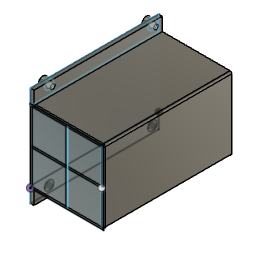
battery_holder v3 (Autodesk Fusion 360 design; units mm, degrees)
Autodesk Fusion 360 part; units mm, degrees
sketch "Sketch1" plane through (0, 0, 0) normal (0, 1, 0) x (1, 0, 0)
  line L0 (0, 0) -> (41, 0)
  line L1 (41, 0) -> (41, -41)
  line L2 (41, -41) -> (0, -41)
  line L3 (0, -41) -> (0, 0)
  line L4 (1, -1) -> (40, -1)
  line L5 (40, -1) -> (40, -40)
  line L6 (40, -40) -> (1, -40)
  line L7 (1, -40) -> (1, -1)
  line L8 (20, -40) -> (20, -1)
  line L9 (21, -40) -> (21, -1)
  line L10 (1, -21) -> (20, -21)
  line L11 (1, -20) -> (20, -20)
  line L12 (21, -21) -> (40, -21)
  line L13 (21, -20) -> (40, -20)
  dimension "d1" = 41
  dimension "d2" = 41
  dimension "d3" = 39
  dimension "d4" = 1
  dimension "d5" = 1
  dimension "d6" = 19
  dimension "d7" = 19
  dimension "d8" = 1
  dimension "d9" = 1
  dimension "d10" = 19
  dimension "d11" = 19
  constraint horizontal L0
  constraint vertical L1
  constraint horizontal L2
  constraint vertical L3
  constraint coincident L0.start L3.end
  constraint horizontal L4
  constraint vertical L5
  constraint horizontal L6
  constraint vertical L7
  constraint coincident L6 L8.start
  constraint coincident L4 L8.end
  constraint perpendicular L4 L8
  constraint coincident L6 L9.start
  constraint coincident L4 L9.end
  constraint perpendicular L4 L9
  constraint coincident L7 L10.start
  constraint coincident L8 L10.end
  constraint perpendicular L8 L10
  constraint coincident L7 L11.start
  constraint coincident L8 L11.end
  constraint perpendicular L7 L11
  constraint coincident L9 L12.start
  constraint coincident L5 L12.end
  constraint perpendicular L5 L12
  constraint coincident L9 L13.start
  constraint perpendicular L9 L13
  measures "d1" distance of L0.start L0.end
  measures "d2" distance of L0.start L2.end
  measures "d3" distance of L4.start L6.end
  measures "d4" distance of L0 L4
  measures "d5" distance of L3 L7
  measures "d6" distance of L7 L8
  measures "d7" distance of L5 L9
  measures "d8" distance of L10 L11
  measures "d9" distance of L12 L13
  measures "d10" distance of L4 L11
  measures "d11" distance of L4 L13
extrude "Extrude1" add sketch "Sketch1" along normal blind 68 contours L4 L6 L8 L9 | L7 L8 L10 L11 | L5 L9 L12 L13
extrude "Extrude2" add sketch "Sketch1" along normal blind 72
extrude "Extrude3" add sketch "Sketch1" along normal blind 2 contours L4 L7 L8 L11 | L4 L5 L9 L13 | L6 L7 L8 L10 | L5 L6 L9 L12
ref_plane "WorkPlane1" through (18, 37, 20.5) normal (1, 0, 0) x (0, 0, -1)
sketch "Sketch6" plane through (18, 0, 0) normal (1, 0, 0) x (0, 1, 0)
  line L0 (72, 40) -> (70.5, 40)
  line L1 (70.5, 40) -> (70.5, 39)
  line L2 (70.5, 39) -> (72, 40)
  line L3 (72, 1) -> (70.5, 1)
  line L4 (70.5, 1) -> (70.5, 2)
  line L5 (70.5, 2) -> (72, 1)
  constraint horizontal L0
  constraint perpendicular L0 L1
  constraint perpendicular L1 L3
  constraint perpendicular L3 L4
extrude "Extrude4" add sketch "Sketch6" along normal blind 5
fillet "Fillet1" radius 1 1 edges at (41, 36, 41)
fillet "Fillet2" radius 1 1 edges at (0, 36, 41)
fillet "Fillet3" radius 1 5 edges at (41, 0, 20) (40.7071, 0, 40.7071) (20.5, 0, 41) (0.2929, 0, 40.7071) (0, 0, 20)
fillet "Fillet4" radius 1 5 edges at (41, 36.5, 0) (40.7071, 0.2929, 0) (20.5, 0, 0) (0.2929, 0.2929, 0) (0, 36.5, 0)
sketch "Sketch8" plane through (0, 0, 0) normal (-1, 0, 0) x (0, -1, 0)
  line L0 (-72, 1) -> (-1, 1)
  line L1 (-1, 1) -> (-1, 40)
  line L2 (-1, 40) -> (-72, 40)
  line L3 (-72, 40) -> (-72, 1)
  line L4 (-72, 1) -> (0, 1)
  line L5 (0, 1) -> (0, -7.5)
  line L6 (0, -7.5) -> (-72, -7.5)
  line L7 (-72, -7.5) -> (-72, 1)
  line L8 (0, 40) -> (-72, 40)
  line L9 (-72, 40) -> (-72, 48.5)
  line L10 (-72, 48.5) -> (0, 48.5)
  line L11 (0, 48.5) -> (0, 40)
  circle A0 centre (-68.5, 45) radius 2.5
  circle A1 centre (-10.5, 45) radius 2.5
  circle A2 centre (-68.5, -4) radius 2.5
  circle A3 centre (-10.5, -4) radius 2.5
  dimension "d41" = 8.5
  dimension "d42" = 8.5
  dimension "d44" = 5
  dimension "d45" = 5
  dimension "d46" = 5
  dimension "d47" = 5
  dimension "d48" = 3.5
  dimension "d49" = 3.5
  dimension "d50" = 3.5
  dimension "d51" = 3.5
  dimension "d52" = 3.5
  dimension "d53" = 3.5
  dimension "d54" = 58
  dimension "d55" = 58
  constraint horizontal L4
  constraint vertical L5
  constraint horizontal L6
  constraint vertical L7
  constraint coincident L0.start L3.end
  constraint horizontal L8
  constraint vertical L9
  constraint horizontal L10
  constraint vertical L11
  measures "d41" distance of L0.start L6.end
  measures "d42" distance of L2.end L9.end
  measures "d44" diameter of A0
  measures "d45" diameter of A1
  measures "d46" diameter of A3
  measures "d47" diameter of A2
  measures "d48" distance of L9 A0.centre
  measures "d49" distance of L10 A0.centre
  measures "d50" distance of L10 A1.centre
  measures "d51" distance of L6 A3.centre
  measures "d52" distance of L7 A2.centre
  measures "d53" distance of L6 A2.centre
  measures "d54" distance of A0.centre A1.centre
  measures "d55" distance of A2.centre A3.centre
extrude "Extrude5" add sketch "Sketch8" along normal blind 0 and the other way blind 2 contours L0 L4 L5 L6 L7 | L2 L8 L9 L10 L11 | A0 | A1 | A2 | A3
extrude "Extrude6" add sketch "Sketch8" along normal blind 3.5 contours A0 | A1 | A2 | A3
hole "Hole1" at (0, 68.5, 45) direction (-1, 0, 0) diameter 2.076 depth 6 tip angle 180
thread "Thread1" "ISO Metric profile 2.5 M2.5x0.45 6H" thread offset 0 thread depth 7.4
hole "Hole2" at (0, 68.5, 45) direction (1, 0, 0) diameter 2.076 depth 2.5 tip angle 180
thread "Thread2" "ISO Metric profile 2.5 M2.5x0.45 6H" thread offset 0 thread depth 7.4
hole "Hole3" at (0, 10.5, 45) direction (1, 0, 0) diameter 2.076 depth 11 tip angle 180
thread "Thread3" "ISO Metric profile 2.5 M2.5x0.45 6H" thread offset 0 thread depth 7.4
hole "Hole4" at (0, 10.5, 45) direction (-1, 0, 0) diameter 2.076 depth 11 tip angle 180
thread "Thread4" "ISO Metric profile 2.5 M2.5x0.45 6H" thread offset 0 thread depth 7.4
hole "Hole5" at (0, 10.5, -4) direction (1, 0, 0) diameter 2.076 depth 9 tip angle 180
thread "Thread5" "ISO Metric profile 2.5 M2.5x0.45 6H" thread offset 0 thread depth 7.4
hole "Hole6" at (0, 10.5, -4) direction (-1, 0, 0) diameter 2.076 depth 9 tip angle 180
thread "Thread6" "ISO Metric profile 2.5 M2.5x0.45 6H" thread offset 0 thread depth 7.4
hole "Hole7" at (0, 68.5, -4) direction (1, 0, 0) diameter 2.076 depth 9 tip angle 180
thread "Thread7" "ISO Metric profile 2.5 M2.5x0.45 6H" thread offset 0 thread depth 7.4
hole "Hole8" at (0, 68.5, -4) direction (-1, 0, 0) diameter 2.076 depth 9 tip angle 180
thread "Thread8" "ISO Metric profile 2.5 M2.5x0.45 6H" thread offset 0 thread depth 7.4
hole "Hole9" at (0, 68.5, 45) at (0, 10.5, 45) at (0, 10.5, -4) at (0, 68.5, -4) direction (-1, 0, 0) diameter 2.529 end through all
thread "Thread9" "ISO Metric profile 3.0 M3x0.5 6H" thread offset 0 thread depth 7.4
hole "Hole10" at (0, 10.5, 45) at (0, 68.5, 45) at (0, 10.5, -4) at (0, 68.5, -4) direction (1, 0, 0) diameter 2.529 depth 6 tip angle 180
thread "Thread10" "ISO Metric profile 3.0 M3x0.5 6H" thread offset 0 thread depth 7.4
